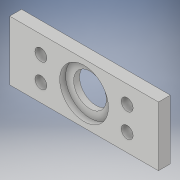
# Autodesk Inventor part: bottom
Saved by Autodesk Inventor 2019 (Build 230136000, 136)
## iProperties
Created: 2018-08-03
Part Number: bottom
Material: Generic
Document SubType Name: Modeling
Designer: Brian
Density: 1 g/cm^3
Appearance: Default
Author: Brian
Autodesk Inventor part; units mm, degrees
ref_plane "YZ Plane" through (0, 0, 0) normal (1, 0, 0) x (0, 1, 0)
ref_plane "XZ Plane" through (0, 0, 0) normal (0, 1, 0) x (-1, 0, 0)
ref_plane "XY Plane" through (0, 0, 0) normal (0, 0, 1) x (1, 0, 0)
sketch "Sketch1" plane through (0, 0, 0) normal (0, 0, 1) x (1, 0, 0)
  line L0 (0, 0) -> (50, 0)
  line L1 (50, 0) -> (50, 20)
  line L2 (50, 20) -> (0, 20)
  line L3 (0, 20) -> (0, 0)
  dimension "d0" = 50
  dimension "d1" = 20
  constraints: 8 end point, 2 parallel, 1 horizontal, 1 perpendicular
  measures "d0" distance of L2.end L1.end
  measures "d1" distance of L1.end L0.end
extrude "Extrusion1" add sketch "Sketch1" along normal blind 4
sketch "Sketch2" plane through (0, 0, 4) normal (0, 0, 1) x (1, 0, 0)
  line L0 (50, 20) -> (0, 20) projected
  line L1 (0, 20) -> (0, 0) projected
  point P0 (25, 10)
  dimension "d11" = 10
  dimension "d12" = 25
  measures "d11" distance from line of L0 point (25, 10)
  measures "d12" distance from line of L1 point (25, 10)
hole "Hole1" at (25, 10, 4) direction (0, 0, -1) diameter 11 depth 4 tip angle 118 counterbore diameter 16.4 counterbore depth 2
sketch "Sketch3" plane through (0, 0, 4) normal (0, 0, 1) x (1, 0, 0)
  line L0 (50, 0) -> (50, 20) projected
  line L1 (50, 20) -> (0, 20) projected
  point P0 (0, 0)
  point P1 (39.5, 14.0277)
  dimension "d21" = 10.5
  dimension "d22" = 5.9723
  measures "d21" distance from line of L0 point (39.5, 14.028)
  measures "d22" distance from line of L1 point (39.5, 14.028)
hole "Hole2" at (39.5, 14.0277, 4) direction (0, 0, -1) diameter 4 end through all
sketch "Sketch4" plane through (0, 0, 4) normal (0, 0, 1) x (1, 0, 0)
  line L0 (0, 0) -> (50, 0) projected
  line L1 (50, 0) -> (50, 20) projected
  point P0 (39.5, 5.9723)
  dimension "d30" = 5.9723
  dimension "d31" = 10.5
  measures "d30" distance from line of L0 point (39.5, 5.972)
  measures "d31" distance from line of L1 point (39.5, 5.972)
hole "Hole3" at (39.5, 5.9723, 4) direction (0, 0, -1) diameter 4 end through all
sketch "Sketch5" plane through (0, 0, 4) normal (0, 0, 1) x (1, 0, 0)
  line L0 (50, 20) -> (0, 20) projected
  line L1 (0, 20) -> (0, 0) projected
  point P0 (10.5, 14.0277)
  dimension "d46" = 5.9723
  dimension "d47" = 10.5
  measures "d46" distance from line of L0 point (10.5, 14.028)
  measures "d47" distance from line of L1 point (10.5, 14.028)
hole "Hole4" at (10.5, 14.0277, 4) direction (0, 0, -1) diameter 4 end through all
sketch "Sketch6" plane through (0, 0, 4) normal (0, 0, 1) x (1, 0, 0)
  line L0 (0, 20) -> (0, 0) projected
  line L1 (0, 0) -> (50, 0) projected
  point P0 (10.5, 5.9723)
  dimension "d48" = 10.5
  dimension "d49" = 5.9723
  measures "d48" distance from line of L0 point (10.5, 5.972)
  measures "d49" distance from line of L1 point (10.5, 5.972)
hole "Hole5" at (10.5, 5.9723, 4) direction (0, 0, -1) diameter 4 end through all
body "Solid1"
